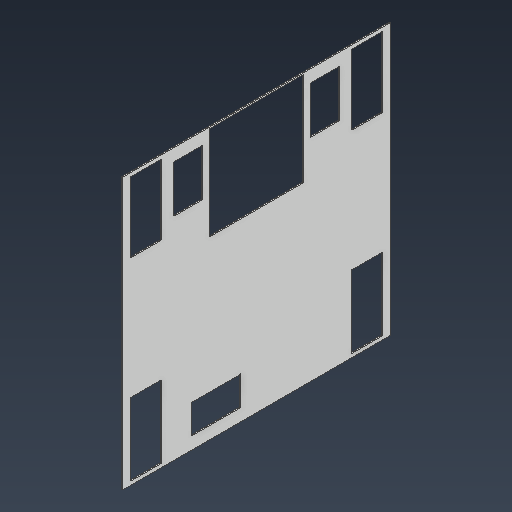
# Autodesk Inventor part: дно 25-26
Saved by Autodesk Inventor 2025.2 (Build 292293000, 293)
## iProperties
Created: 2025-09-06
Part Number: дно 25-26
Material: Типовые
Document SubType Name: Modeling
Designer: Trene
Density: 1 g/cm^3
Appearance: По умолчанию
Author: Trene
Autodesk Inventor part; units mm, degrees
ref_plane "YZ Plane" through (0, 0, 0) normal (1, 0, 0) x (0, 1, 0)
ref_plane "XZ Plane" through (0, 0, 0) normal (0, 1, 0) x (-1, 0, 0)
ref_plane "XY Plane" through (0, 0, 0) normal (0, 0, 1) x (1, 0, 0)
sketch "Эскиз1" plane through (0, 0, 0) normal (1, 0, 0) x (0, 1, 0)
  line L0 (0, 0) -> (370, 0)
  line L1 (370, 0) -> (370, -370)
  line L2 (370, -370) -> (0, -370)
  line L3 (0, -370) -> (0, 0)
  dimension "d0" = 370
  dimension "d1" = 370
  constraints: 8 end point, 2 parallel, 1 horizontal, 1 perpendicular
  measures "d0" distance of L1.end L2.end
  measures "d1" distance of L0.end L1.end
extrude "Выдавливание1" add sketch "Эскиз1" along normal blind 1.5
sketch "Эскиз3" plane through (1.5, 0, 0) normal (1, 0, 0) x (0, 0, -1)
  line L0 (0, 0) -> (370, 0) projected
  line L1 (11.25, 0) -> (53.25, 0)
  line L2 (53.25, 0) -> (53.25, 100)
  line L3 (53.25, 100) -> (11.25, 100)
  line L4 (11.25, 100) -> (11.25, 0)
  line L5 (0, 370) -> (0, 0) projected
  line L6 (370, 370) -> (0, 370) projected
  line L7 (185, 370) -> (185, 0)
  line L8 (0, 185) -> (370, 185)
  line L9 (370, 0) -> (370, 370) projected
  line L10 (358.75, 0) -> (316.75, 0)
  line L11 (316.75, 0) -> (316.75, 100)
  line L12 (316.75, 100) -> (358.75, 100)
  line L13 (358.75, 100) -> (358.75, 0)
  line L14 (11.25, 370) -> (53.25, 370)
  line L15 (53.25, 370) -> (53.25, 270)
  line L16 (53.25, 270) -> (11.25, 270)
  line L17 (11.25, 270) -> (11.25, 370)
  line L18 (358.75, 370) -> (316.75, 370)
  line L19 (316.75, 370) -> (316.75, 270)
  line L20 (316.75, 270) -> (358.75, 270)
  line L21 (358.75, 270) -> (358.75, 370)
  point P0 (358.75, 370)
  point P1 (11.25, 370)
  dimension "d9" = 42
  dimension "d10" = 100
  dimension "d13" = 11.25
  constraints: 36 end point, 12 symmetric about line, 4 midpoint, 2 parallel, 1 horizontal, 1 perpendicular, 1 point on line
  measures "d9" distance of L3.end L2.end
  measures "d10" distance of L2.end L1.end
  measures "d13" distance between parallel lines of L5 L4
extrude "Выдавливание3" cut sketch "Эскиз3" against normal blind 10 contours L4 L3 L2 L0 | L6 L15 L16 L17 | L11 L12 L13 L0 | L6 L21 L20 L19
sketch "Эскиз4" plane through (1.5, 0, 0) normal (1, 0, 0) x (0, 0, -1)
  line L0 (53.25, 0) -> (316.75, 0) projected
  line L1 (185, 0) -> (185, 257.6138)
  line L2 (0, 370) -> (0, 0) projected
  line L3 (0, 185) -> (403.9864, 185)
  line L4 (120, 370.5966) -> (250, 370.5966)
  line L5 (250, 370.5966) -> (250, 240.5966)
  line L6 (250, 240.5966) -> (120, 240.5966)
  line L7 (120, 240.5966) -> (120, 370.5966)
  line L8 (120, 370.5966) -> (250, 240.5966) construction
  line L9 (250, 370.5966) -> (120, 240.5966) construction
  point P0 (185, 370)
  point P1 (185, 305.5966)
  constraints: 16 end point, 2 midpoint, 1 horizontal, 1 symmetric about line, 1 vertical
extrude "Выдавливание4" cut sketch "Эскиз4" against normal blind 10
sketch "Эскиз5" plane through (1.5, 0, 0) normal (1, 0, 0) x (0, 0, -1)
  line L0 (250, 370) -> (299, 370)
  line L1 (316.75, 370) -> (250, 370) projected
  line L2 (299, 370) -> (259, 370)
  line L3 (259, 370) -> (259, 290)
  line L4 (259, 290) -> (299, 290)
  line L5 (299, 290) -> (299, 370)
  line L6 (53.25, 0) -> (316.75, 0) projected
  line L7 (185, 0) -> (185, 405.4433)
  line L8 (71, 370) -> (111, 370)
  line L9 (111, 370) -> (111, 290)
  line L10 (111, 290) -> (71, 290)
  line L11 (71, 290) -> (71, 370)
  line L12 (53.25, 100) -> (53.25, 0) projected
  line L13 (53.25, 0) -> (95.25, 0)
  line L14 (53.25, 0) -> (163.25, 0)
  line L15 (163.25, 0) -> (163.25, 55)
  line L16 (163.25, 55) -> (53.25, 55)
  line L17 (53.25, 55) -> (53.25, 0)
  line L18 (95.25, 0) -> (95.25, 55)
  line L19 (316.75, 100) -> (358.75, 100) projected
  line L20 (316.75, 100) -> (358.75, 100)
  line L21 (358.75, 100) -> (358.75, 103)
  line L22 (358.75, 103) -> (316.75, 103)
  line L23 (316.75, 103) -> (316.75, 100)
  line L24 (53.25, 100) -> (11.25, 100)
  line L25 (53.25, 100) -> (11.25, 100)
  line L26 (11.25, 100) -> (11.25, 103)
  line L27 (11.25, 103) -> (53.25, 103)
  line L28 (53.25, 103) -> (53.25, 100)
  point P0 (0, 0)
  point P1 (53.25, 55)
  point P2 (163.25, 0)
  dimension "d20" = 49
  dimension "d21" = 40
  dimension "d22" = 80
  dimension "d25" = 42
  dimension "d26" = 110
  dimension "d27" = 55
  dimension "d36" = 42
  dimension "d37" = 3
  constraints: 50 end point, 8 symmetric about line, 6 parallel, 3 horizontal, 3 perpendicular, 3 point on line, 2 vertical, 1 midpoint
  measures "d20" distance of L0.start L0.end
  measures "d21" distance of L4.end L3.end
  measures "d22" distance of L3.end L2.end
  measures "d25" distance of L6.start L13.end
  measures "d26" distance of L16.end L15.end
  measures "d27" distance of L15.end L14.end
  measures "d36" distance of L22.end L21.end
  measures "d37" distance of L21.end L20.end
extrude "Выдавливание5" cut sketch "Эскиз5" against normal blind 10 contours L0 L5 L4 L3 | L18 L16 L15 L6 | L8 L9 L10 L11 | L23 L22 L21 L19 | L24 L26 L27 L28
sketch "Эскиз6" plane through (1.5, 0, 0) normal (1, 0, 0) x (0, 0, -1)
  line L0 (316.75, 370) -> (299, 370) projected
  line L1 (299, 370) -> (259, 370)
  line L2 (259, 370) -> (259, 355)
  line L3 (259, 355) -> (299, 355)
  line L4 (299, 355) -> (299, 370)
  line L5 (250, 240.5966) -> (120, 240.5966) projected
  line L6 (185, 240.5966) -> (185, 152.8583)
  line L7 (71, 370) -> (111, 370)
  line L8 (111, 370) -> (111, 355)
  line L9 (111, 355) -> (71, 355)
  line L10 (71, 355) -> (71, 370)
  line L11 (95.25, 0) -> (95.25, 55) projected
  line L12 (95.25, 0) -> (163.25, 0)
  line L13 (163.25, 0) -> (163.25, 15)
  line L14 (163.25, 15) -> (95.25, 15)
  line L15 (95.25, 15) -> (95.25, 0)
  line L16 (11.25, 0) -> (53.25, 0)
  line L17 (53.25, 0) -> (53.25, 3)
  line L18 (53.25, 3) -> (11.25, 3)
  line L19 (11.25, 3) -> (11.25, 0)
  line L20 (358.75, 0) -> (316.75, 0)
  line L21 (316.75, 0) -> (316.75, 3)
  line L22 (316.75, 3) -> (358.75, 3)
  line L23 (358.75, 3) -> (358.75, 0)
  line L24 (370, 0) -> (370, 370) projected
  line L25 (370, 0) -> (0, 0)
  line L26 (0, 0) -> (0, -2)
  line L27 (0, -2) -> (370, -2)
  line L28 (370, -2) -> (370, 0)
  line L29 (0, 370) -> (0, 0) projected
  line L30 (0, 185) -> (370, 185)
  line L31 (370, 370) -> (0, 370)
  line L32 (0, 370) -> (0, 372)
  line L33 (0, 372) -> (370, 372)
  line L34 (370, 372) -> (370, 370)
  line L35 (53.25, 370) -> (53.25, 367)
  line L36 (53.25, 367) -> (11.25, 367)
  line L37 (11.25, 367) -> (11.25, 370)
  line L38 (316.75, 370) -> (316.75, 367)
  line L39 (316.75, 367) -> (358.75, 367)
  line L40 (358.75, 367) -> (358.75, 370)
  dimension "d28" = 40
  dimension "d29" = 15
  dimension "d32" = 68
  dimension "d33" = 15
  dimension "d34" = 42
  dimension "d35" = 3
  dimension "d38" = 370
  dimension "d39" = 2
  constraints: 72 end point, 18 symmetric about line, 8 parallel, 4 horizontal, 4 perpendicular, 3 midpoint, 1 vertical
  measures "d28" distance of L3.end L2.end
  measures "d29" distance of L2.end L1.end
  measures "d32" distance of L14.end L13.end
  measures "d33" distance of L13.end L12.end
  measures "d34" distance of L18.end L17.end
  measures "d35" distance of L17.end L16.end
  measures "d38" distance of L27.end L26.end
  measures "d39" distance of L26.end L25.end
extrude "Выдавливание6" add sketch "Эскиз6" against normal up to surface (1.5 mm away) contours L0 L1 L31 L7 L32 L33 L34 | L31 L40 L39 L38 | L4 L3 L2 L1 | L8 L9 L10 L7 | L28 L27 L26 L25 L16 L12 L20 | L35 L36 L37 L31 | L20 L21 L22 L23 | L12 L11 L14 L13 | L19 L18 L17 L16
